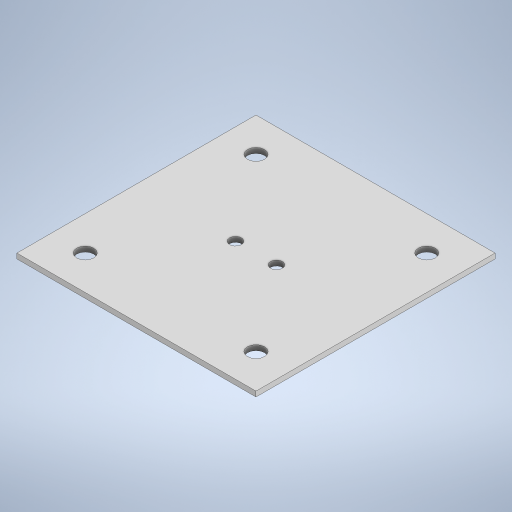
# Autodesk Inventor part: Пластина
Saved by Autodesk Inventor 2023 (Build 270158000, 158)
## iProperties
Created: 2022-05-06
Part Number: Пластина
Material: Типовые
Document SubType Name: Modeling
Designer: avkap
Density: 1 g/cm^3
Appearance: По умолчанию
Author: avkap
Autodesk Inventor part; units mm, degrees
ref_plane "YZ Plane" through (0, 0, 0) normal (1, 0, 0) x (0, 1, 0)
ref_plane "XZ Plane" through (0, 0, 0) normal (0, 1, 0) x (-1, 0, 0)
ref_plane "XY Plane" through (0, 0, 0) normal (0, 0, 1) x (1, 0, 0)
sketch "Эскиз1" plane through (0, 0, 0) normal (0, 1, 0) x (-1, 0, 0)
  line L0 (0, 0) -> (-140, 0)
  line L1 (-140, 0) -> (-140, -140)
  line L2 (-140, -140) -> (0, -140)
  line L3 (0, -140) -> (0, 0)
  line L4 (0, 0) -> (-20, 0)
  line L5 (-20, 0) -> (-20, -20)
  line L6 (-20, -20) -> (0, -20)
  line L7 (0, -20) -> (0, 0)
  line L8 (-140, -140) -> (-120, -140)
  line L9 (-120, -140) -> (-120, -120)
  line L10 (-120, -120) -> (-140, -120)
  line L11 (-140, -120) -> (-140, -140)
  line L12 (-120, -120) -> (-20, -120)
  line L13 (-20, -120) -> (-20, -20)
  line L14 (-20, -20) -> (-120, -20)
  line L15 (-120, -20) -> (-120, -120)
  circle A0 centre (-20, -20) radius 5
  circle A1 centre (-20, -120) radius 5
  circle A2 centre (-120, -20) radius 5
  circle A3 centre (-120, -120) radius 5
  line L16 (-140, -70) -> (0, -70)
  line L17 (-70, -70) -> (-58, -70)
  line L18 (-58, -70) -> (-82, -70)
  circle A4 centre (-58, -70) radius 3.5
  circle A5 centre (-82, -70) radius 3.5
  dimension "d0" = 140
  dimension "d1" = 140
  dimension "d2" = 20
  dimension "d3" = 20
  dimension "d4" = 20
  dimension "d5" = 20
  dimension "d6" = 10
  dimension "d7" = 10
  dimension "d8" = 10
  dimension "d9" = 10
  dimension "d10" = 12
  dimension "d11" = 24
  dimension "d12" = 7
  dimension "d13" = 7
  constraints: 38 end point, 8 parallel, 6 centre point, 6 coincident, 4 horizontal, 4 perpendicular, 3 midpoint, 2 point on line
  measures "d0" distance of L2.end L1.end
  measures "d1" distance of L1.end L0.end
  measures "d2" distance of L6.end L5.end
  measures "d3" distance of L5.end L4.end
  measures "d4" distance of L10.end L9.end
  measures "d5" distance of L9.end L8.end
  measures "d6" diameter of A0
  measures "d7" diameter of A1
  measures "d8" diameter of A2
  measures "d9" diameter of A3
  measures "d10" distance of L17.start L17.end
  measures "d11" distance of L17.end L18.end
  measures "d12" diameter of A4
  measures "d13" diameter of A5
extrude "Выдавливание1" add sketch "Эскиз1" along normal blind 3 contours L3 L6 A0 L5 L0 | L5 A0 L14 A2 L15 L16 L1 L0 | L3 L16 L13 A0 L6 | L3 L2 L9 A3 L12 A1 L13 L16 | L16 L15 A3 L10 L1 | A0 L13 L16 A4 A5 L15 A2 L14 | L13 A1 L12 A3 L15 L16 A5 A4 | L10 A3 L9 L2 L1
